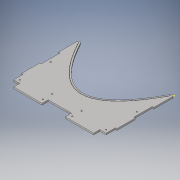
# Autodesk Inventor part: vrRig_v01r1_top
Saved by Autodesk Inventor 2016 (Build 200138000, 138)
## iProperties
Created: 2018-01-13
Part Number: vrRig_v01r1_top
Material: Generic
Document SubType Name: Modeling
Designer: harveylab
Density: 1 g/cm^3
Appearance: Default
Author: harveylab
Autodesk Inventor part; units mm, degrees
ref_plane "YZ Plane" through (0, 0, 0) normal (1, 0, 0) x (0, 1, 0)
ref_plane "XZ Plane" through (0, 0, 0) normal (0, 1, 0) x (-1, 0, 0)
ref_plane "XY Plane" through (0, 0, 0) normal (0, 0, 1) x (1, 0, 0)
sketch "Sketch1" plane through (0, 0, 0) normal (0, 1, 0) x (-1, 0, 0)
  circle A0 centre (374.65, 134.145) radius 3.302 construction
  line L0 (387.3499, 6.3502) -> (384.81, 11.082)
  line L1 (384.81, 11.082) -> (382.27, 15.7505)
  line L2 (382.27, 15.7505) -> (379.73, 20.353)
  line L3 (379.73, 20.353) -> (377.19, 24.8945)
  line L4 (377.19, 24.8945) -> (374.65, 29.37)
  line L5 (374.65, 29.37) -> (372.11, 33.7833)
  line L6 (372.11, 33.7833) -> (369.57, 38.133)
  line L7 (369.57, 38.133) -> (367.03, 42.4193)
  line L8 (367.03, 42.4193) -> (364.49, 46.642)
  line L9 (364.49, 46.642) -> (361.95, 50.8013)
  line L10 (361.95, 50.8013) -> (359.41, 54.897)
  line L11 (359.41, 54.897) -> (356.87, 58.9293)
  line L12 (356.87, 58.9293) -> (354.33, 62.898)
  line L13 (354.33, 62.898) -> (351.79, 66.8033)
  line L14 (351.79, 66.8033) -> (349.25, 70.645)
  line L15 (349.25, 70.645) -> (346.71, 74.4233)
  line L16 (346.71, 74.4233) -> (344.17, 78.138)
  line L17 (344.17, 78.138) -> (341.63, 81.7893)
  line L18 (341.63, 81.7893) -> (339.09, 85.377)
  line L19 (339.09, 85.377) -> (336.55, 88.9025)
  line L20 (336.55, 88.9025) -> (334.01, 92.362)
  line L21 (334.01, 92.362) -> (331.47, 95.7605)
  line L22 (331.47, 95.7605) -> (328.93, 99.093)
  line L23 (328.93, 99.093) -> (326.39, 102.3645)
  line L24 (326.39, 102.3645) -> (323.85, 105.57)
  line L25 (323.85, 105.57) -> (321.31, 108.712)
  line L26 (321.31, 108.712) -> (318.77, 111.793)
  line L27 (318.77, 111.793) -> (316.23, 114.8105)
  line L28 (316.23, 114.8105) -> (313.69, 117.762)
  line L29 (313.69, 117.762) -> (311.15, 120.6525)
  line L30 (311.15, 120.6525) -> (308.61, 123.477)
  line L31 (308.61, 123.477) -> (306.07, 126.2405)
  line L32 (306.07, 126.2405) -> (303.53, 128.938)
  line L33 (303.53, 128.938) -> (300.99, 131.5745)
  line L34 (300.99, 131.5745) -> (298.45, 134.145)
  line L35 (298.45, 134.145) -> (295.91, 136.652)
  line L36 (295.91, 136.652) -> (293.37, 139.098)
  line L37 (293.37, 139.098) -> (290.83, 141.478)
  line L38 (290.83, 141.478) -> (288.29, 143.797)
  line L39 (288.29, 143.797) -> (285.75, 146.0525)
  line L40 (285.75, 146.0525) -> (283.21, 148.242)
  line L41 (283.21, 148.242) -> (280.67, 150.368)
  line L42 (280.67, 150.368) -> (278.13, 152.433)
  line L43 (278.13, 152.433) -> (275.59, 154.4345)
  line L44 (275.59, 154.4345) -> (273.05, 156.37)
  line L45 (273.05, 156.37) -> (270.51, 158.2445)
  line L46 (270.51, 158.2445) -> (267.97, 160.053)
  line L47 (267.97, 160.053) -> (265.43, 161.8005)
  line L48 (265.43, 161.8005) -> (262.89, 163.482)
  line L49 (262.89, 163.482) -> (260.35, 165.1025)
  line L50 (260.35, 165.1025) -> (257.81, 166.657)
  line L51 (257.81, 166.657) -> (255.27, 168.1505)
  line L52 (255.27, 168.1505) -> (252.73, 169.578)
  line L53 (252.73, 169.578) -> (250.19, 170.9445)
  line L54 (250.19, 170.9445) -> (247.65, 172.245)
  line L55 (247.65, 172.245) -> (245.11, 173.4845)
  line L56 (245.11, 173.4845) -> (242.57, 174.658)
  line L57 (242.57, 174.658) -> (240.03, 175.768)
  line L58 (240.03, 175.768) -> (237.49, 176.817)
  line L59 (237.49, 176.817) -> (234.95, 177.8025)
  line L60 (234.95, 177.8025) -> (232.41, 178.722)
  line L61 (232.41, 178.722) -> (229.87, 179.5805)
  line L62 (229.87, 179.5805) -> (227.33, 180.373)
  line L63 (227.33, 180.373) -> (224.79, 181.102)
  line L64 (224.79, 181.102) -> (222.25, 181.77)
  line L65 (222.25, 181.77) -> (219.71, 182.372)
  line L66 (219.71, 182.372) -> (217.17, 182.913)
  line L67 (217.17, 182.913) -> (214.63, 183.388)
  line L68 (214.63, 183.388) -> (212.09, 183.802)
  line L69 (212.09, 183.802) -> (209.55, 184.1525)
  line L70 (209.55, 184.1525) -> (207.01, 184.437)
  line L71 (207.01, 184.437) -> (204.47, 184.658)
  line L72 (204.47, 184.658) -> (201.93, 184.818)
  line L73 (201.93, 184.818) -> (199.39, 184.9145)
  line L74 (199.39, 184.9145) -> (196.85, 184.945)
  line L75 (381.755, 3.3486) -> (379.2235, 8.0648)
  line L76 (379.2235, 8.0648) -> (376.7012, 12.7009)
  line L77 (376.7012, 12.7009) -> (374.1791, 17.2709)
  line L78 (374.1791, 17.2709) -> (371.6575, 21.7794)
  line L79 (371.6575, 21.7794) -> (369.1368, 26.2209)
  line L80 (369.1368, 26.2209) -> (366.6163, 30.6003)
  line L81 (366.6163, 30.6003) -> (364.0967, 34.9152)
  line L82 (364.0967, 34.9152) -> (361.5777, 39.1659)
  line L83 (361.5777, 39.1659) -> (359.0595, 43.3525)
  line L84 (359.0595, 43.3525) -> (356.5419, 47.475)
  line L85 (356.5419, 47.475) -> (354.0252, 51.5332)
  line L86 (354.0252, 51.5332) -> (351.5092, 55.5273)
  line L87 (351.5092, 55.5273) -> (348.9941, 59.4572)
  line L88 (348.9941, 59.4572) -> (346.4798, 63.3229)
  line L89 (346.4798, 63.3229) -> (343.9665, 67.1244)
  line L90 (343.9665, 67.1244) -> (341.454, 70.8616)
  line L91 (341.454, 70.8616) -> (338.9426, 74.5346)
  line L92 (338.9426, 74.5346) -> (336.4321, 78.1433)
  line L93 (336.4321, 78.1433) -> (333.9225, 81.6883)
  line L94 (333.9225, 81.6883) -> (331.4145, 85.1693)
  line L95 (331.4145, 85.1693) -> (328.9074, 88.584)
  line L96 (328.9074, 88.584) -> (326.4015, 91.9369)
  line L97 (326.4015, 91.9369) -> (323.8968, 95.223)
  line L98 (323.8968, 95.223) -> (321.3935, 98.4473)
  line L99 (321.3935, 98.4473) -> (318.8923, 101.6039)
  line L100 (318.8923, 101.6039) -> (316.3909, 104.698)
  line L101 (316.3909, 104.698) -> (313.891, 107.7305)
  line L102 (313.891, 107.7305) -> (311.3942, 110.6966)
  line L103 (311.3942, 110.6966) -> (308.8983, 113.5969)
  line L104 (308.8983, 113.5969) -> (306.404, 116.4354)
  line L105 (306.404, 116.4354) -> (303.9114, 119.2072)
  line L106 (303.9114, 119.2072) -> (301.4206, 121.9171)
  line L107 (301.4206, 121.9171) -> (298.9317, 124.5603)
  line L108 (298.9317, 124.5603) -> (296.4448, 127.1417)
  line L109 (296.4448, 127.1417) -> (293.961, 129.6553)
  line L110 (293.961, 129.6553) -> (291.4771, 132.107)
  line L111 (291.4771, 132.107) -> (288.9965, 134.4958)
  line L112 (288.9965, 134.4958) -> (286.5181, 136.818)
  line L113 (286.5181, 136.818) -> (284.0408, 139.0798)
  line L114 (284.0408, 139.0798) -> (281.5685, 141.2752)
  line L115 (281.5685, 141.2752) -> (279.0989, 143.404)
  line L116 (279.0989, 143.404) -> (276.629, 145.4713)
  line L117 (276.629, 145.4713) -> (274.1617, 147.4772)
  line L118 (274.1617, 147.4772) -> (271.7002, 149.4169)
  line L119 (271.7002, 149.4169) -> (269.2401, 151.2915)
  line L120 (269.2401, 151.2915) -> (266.7828, 153.105)
  line L121 (266.7828, 153.105) -> (264.3286, 154.8524)
  line L122 (264.3286, 154.8524) -> (261.8774, 156.5388)
  line L123 (261.8774, 156.5388) -> (259.4294, 158.1594)
  line L124 (259.4294, 158.1594) -> (256.9846, 159.7192)
  line L125 (256.9846, 159.7192) -> (254.543, 161.2134)
  line L126 (254.543, 161.2134) -> (252.1048, 162.6471)
  line L127 (252.1048, 162.6471) -> (249.6699, 164.0155)
  line L128 (249.6699, 164.0155) -> (247.2384, 165.3236)
  line L129 (247.2384, 165.3236) -> (244.8103, 166.5668)
  line L130 (244.8103, 166.5668) -> (242.3856, 167.7501)
  line L131 (242.3856, 167.7501) -> (239.9667, 168.8676)
  line L132 (239.9667, 168.8676) -> (237.5463, 169.9253)
  line L133 (237.5463, 169.9253) -> (235.1292, 170.9236)
  line L134 (235.1292, 170.9236) -> (232.7205, 171.8582)
  line L135 (232.7205, 171.8582) -> (230.3123, 172.7299)
  line L136 (230.3123, 172.7299) -> (227.9074, 173.5428)
  line L137 (227.9074, 173.5428) -> (225.5082, 174.2913)
  line L138 (225.5082, 174.2913) -> (223.1063, 174.9807)
  line L139 (223.1063, 174.9807) -> (220.71, 175.6109)
  line L140 (220.71, 175.6109) -> (218.3161, 176.1783)
  line L141 (218.3161, 176.1783) -> (215.9247, 176.6876)
  line L142 (215.9247, 176.6876) -> (213.5354, 177.1344)
  line L143 (213.5354, 177.1344) -> (211.145, 177.5241)
  line L144 (211.145, 177.5241) -> (208.7624, 177.8529)
  line L145 (208.7624, 177.8529) -> (206.3813, 178.1196)
  line L146 (206.3813, 178.1196) -> (203.9951, 178.3272)
  line L147 (203.9951, 178.3272) -> (201.6097, 178.4774)
  line L148 (201.6097, 178.4774) -> (199.2313, 178.5678)
  line L149 (199.2313, 178.5678) -> (196.9262, 178.5955)
  line L150 (386.6786, 5.9898) -> (384.1396, 10.72)
  line L151 (384.1396, 10.72) -> (381.6018, 15.3846)
  line L152 (381.6018, 15.3846) -> (379.0639, 19.9832)
  line L153 (379.0639, 19.9832) -> (376.5261, 24.5207)
  line L154 (376.5261, 24.5207) -> (373.9884, 28.9921)
  line L155 (373.9884, 28.9921) -> (371.4508, 33.4013)
  line L156 (371.4508, 33.4013) -> (368.9132, 37.7469)
  line L157 (368.9132, 37.7469) -> (366.3757, 42.0289)
  line L158 (366.3757, 42.0289) -> (363.8384, 46.2473)
  line L159 (363.8384, 46.2473) -> (361.3011, 50.4021)
  line L160 (361.3011, 50.4021) -> (358.7638, 54.4934)
  line L161 (358.7638, 54.4934) -> (356.2267, 58.521)
  line L162 (356.2267, 58.521) -> (353.6897, 62.4851)
  line L163 (353.6897, 62.4851) -> (351.1528, 66.3856)
  line L164 (351.1528, 66.3856) -> (348.616, 70.2225)
  line L165 (348.616, 70.2225) -> (346.0793, 73.9959)
  line L166 (346.0793, 73.9959) -> (343.5427, 77.7056)
  line L167 (343.5427, 77.7056) -> (341.0063, 81.3518)
  line L168 (341.0063, 81.3518) -> (338.4699, 84.9344)
  line L169 (338.4699, 84.9344) -> (335.9338, 88.4545)
  line L170 (335.9338, 88.4545) -> (333.3977, 91.9087)
  line L171 (333.3977, 91.9087) -> (330.8618, 95.3017)
  line L172 (330.8618, 95.3017) -> (328.326, 98.6286)
  line L173 (328.326, 98.6286) -> (325.7904, 101.8945)
  line L174 (325.7904, 101.8945) -> (323.2551, 105.0941)
  line L175 (323.2551, 105.0941) -> (320.7197, 108.2303)
  line L176 (320.7197, 108.2303) -> (318.1845, 111.3055)
  line L177 (318.1845, 111.3055) -> (315.6497, 114.3169)
  line L178 (315.6497, 114.3169) -> (313.115, 117.2622)
  line L179 (313.115, 117.2622) -> (310.5805, 120.1465)
  line L180 (310.5805, 120.1465) -> (308.0462, 122.9646)
  line L181 (308.0462, 122.9646) -> (305.5121, 125.7217)
  line L182 (305.5121, 125.7217) -> (302.9782, 128.4127)
  line L183 (302.9782, 128.4127) -> (300.4446, 131.0426)
  line L184 (300.4446, 131.0426) -> (297.9113, 133.6063)
  line L185 (297.9113, 133.6063) -> (295.3781, 136.1066)
  line L186 (295.3781, 136.1066) -> (292.8452, 138.5457)
  line L187 (292.8452, 138.5457) -> (290.3126, 140.9188)
  line L188 (290.3126, 140.9188) -> (287.7801, 143.2309)
  line L189 (287.7801, 143.2309) -> (285.2482, 145.4793)
  line L190 (285.2482, 145.4793) -> (282.7167, 147.6615)
  line L191 (282.7167, 147.6615) -> (280.1851, 149.7804)
  line L192 (280.1851, 149.7804) -> (277.6538, 151.8383)
  line L193 (277.6538, 151.8383) -> (275.1232, 153.8324)
  line L194 (275.1232, 153.8324) -> (272.5928, 155.7606)
  line L195 (272.5928, 155.7606) -> (270.0628, 157.6278)
  line L196 (270.0628, 157.6278) -> (267.5331, 159.4289)
  line L197 (267.5331, 159.4289) -> (265.0037, 161.1691)
  line L198 (265.0037, 161.1691) -> (262.4747, 162.8433)
  line L199 (262.4747, 162.8433) -> (259.9462, 164.4565)
  line L200 (259.9462, 164.4565) -> (257.418, 166.0038)
  line L201 (257.418, 166.0038) -> (254.8902, 167.4901)
  line L202 (254.8902, 167.4901) -> (252.3628, 168.9105)
  line L203 (252.3628, 168.9105) -> (249.8358, 170.27)
  line L204 (249.8358, 170.27) -> (247.3093, 171.5636)
  line L205 (247.3093, 171.5636) -> (244.7831, 172.7964)
  line L206 (244.7831, 172.7964) -> (242.2576, 173.9632)
  line L207 (242.2576, 173.9632) -> (239.732, 175.0669)
  line L208 (239.732, 175.0669) -> (237.2067, 176.1098)
  line L209 (237.2067, 176.1098) -> (234.6825, 177.0892)
  line L210 (234.6825, 177.0892) -> (232.1583, 178.003)
  line L211 (232.1583, 178.003) -> (229.6345, 178.856)
  line L212 (229.6345, 178.856) -> (227.1114, 179.6432)
  line L213 (227.1114, 179.6432) -> (224.588, 180.3674)
  line L214 (224.588, 180.3674) -> (222.0652, 181.0309)
  line L215 (222.0652, 181.0309) -> (219.5428, 181.6287)
  line L216 (219.5428, 181.6287) -> (217.0206, 182.166)
  line L217 (217.0206, 182.166) -> (214.4987, 182.6376)
  line L218 (214.4987, 182.6376) -> (211.9766, 183.0487)
  line L219 (211.9766, 183.0487) -> (209.4555, 183.3966)
  line L220 (209.4555, 183.3966) -> (206.9346, 183.6789)
  line L221 (206.9346, 183.6789) -> (204.413, 183.8983)
  line L222 (204.413, 183.8983) -> (201.8916, 184.0571)
  line L223 (201.8916, 184.0571) -> (199.371, 184.1529)
  line L224 (199.371, 184.1529) -> (196.8592, 184.1831)
  arc A1 (381.755, 3.3486) -> (393.6991, 6.3502) centre (387.3499, 6.3502) ccw
  line L225 (393.6991, 6.3502) -> (393.6991, 7.1452)
  line L226 (387.3499, 6.3502) -> (386.6786, 5.9898)
  line L227 (393.6991, 7.1452) -> (393.6991, 83.3452)
  line L228 (393.6991, 83.3452) -> (387.3491, 83.3452)
  line L229 (387.3491, 83.3452) -> (387.3491, 159.5452)
  line L230 (387.3491, 159.5452) -> (393.6991, 159.5452)
  line L231 (393.6991, 159.5452) -> (393.6991, 235.745)
  line L232 (393.6991, 235.745) -> (387.35, 235.745)
  line L233 (387.35, 235.745) -> (387.35, 273.845)
  circle A2 centre (19.05, 134.145) radius 3.302 construction
  line L234 (6.35, 6.35) -> (8.89, 11.082)
  line L235 (8.89, 11.082) -> (11.43, 15.7505)
  line L236 (11.43, 15.7505) -> (13.97, 20.353)
  line L237 (13.97, 20.353) -> (16.51, 24.8945)
  line L238 (16.51, 24.8945) -> (19.05, 29.37)
  line L239 (19.05, 29.37) -> (21.59, 33.7833)
  line L240 (21.59, 33.7833) -> (24.13, 38.133)
  line L241 (24.13, 38.133) -> (26.67, 42.4193)
  line L242 (26.67, 42.4193) -> (29.21, 46.642)
  line L243 (29.21, 46.642) -> (31.75, 50.8013)
  line L244 (31.75, 50.8013) -> (34.29, 54.897)
  line L245 (34.29, 54.897) -> (36.83, 58.9293)
  line L246 (36.83, 58.9293) -> (39.37, 62.898)
  line L247 (39.37, 62.898) -> (41.91, 66.8033)
  line L248 (41.91, 66.8033) -> (44.45, 70.645)
  line L249 (44.45, 70.645) -> (46.99, 74.4233)
  line L250 (46.99, 74.4233) -> (49.53, 78.138)
  line L251 (49.53, 78.138) -> (52.07, 81.7893)
  line L252 (52.07, 81.7893) -> (54.61, 85.377)
  line L253 (54.61, 85.377) -> (57.15, 88.9025)
  line L254 (57.15, 88.9025) -> (59.69, 92.362)
  line L255 (59.69, 92.362) -> (62.23, 95.7605)
  line L256 (62.23, 95.7605) -> (64.77, 99.093)
  line L257 (64.77, 99.093) -> (67.31, 102.3645)
  line L258 (67.31, 102.3645) -> (69.85, 105.57)
  line L259 (69.85, 105.57) -> (72.39, 108.712)
  line L260 (72.39, 108.712) -> (74.93, 111.793)
  line L261 (74.93, 111.793) -> (77.47, 114.8105)
  line L262 (77.47, 114.8105) -> (80.01, 117.762)
  line L263 (80.01, 117.762) -> (82.55, 120.6525)
  line L264 (82.55, 120.6525) -> (85.09, 123.477)
  line L265 (85.09, 123.477) -> (87.63, 126.2405)
  line L266 (87.63, 126.2405) -> (90.17, 128.938)
  line L267 (90.17, 128.938) -> (92.71, 131.5745)
  line L268 (92.71, 131.5745) -> (95.25, 134.145)
  line L269 (95.25, 134.145) -> (97.79, 136.652)
  line L270 (97.79, 136.652) -> (100.33, 139.098)
  line L271 (100.33, 139.098) -> (102.87, 141.478)
  line L272 (102.87, 141.478) -> (105.41, 143.797)
  line L273 (105.41, 143.797) -> (107.95, 146.0525)
  line L274 (107.95, 146.0525) -> (110.49, 148.242)
  line L275 (110.49, 148.242) -> (113.03, 150.368)
  line L276 (113.03, 150.368) -> (115.57, 152.433)
  line L277 (115.57, 152.433) -> (118.11, 154.4345)
  line L278 (118.11, 154.4345) -> (120.65, 156.37)
  line L279 (120.65, 156.37) -> (123.19, 158.2445)
  line L280 (123.19, 158.2445) -> (125.73, 160.053)
  line L281 (125.73, 160.053) -> (128.27, 161.8005)
  line L282 (128.27, 161.8005) -> (130.81, 163.482)
  line L283 (130.81, 163.482) -> (133.35, 165.1025)
  line L284 (133.35, 165.1025) -> (135.89, 166.657)
  line L285 (135.89, 166.657) -> (138.43, 168.1505)
  line L286 (138.43, 168.1505) -> (140.97, 169.578)
  line L287 (140.97, 169.578) -> (143.51, 170.9445)
  line L288 (143.51, 170.9445) -> (146.05, 172.245)
  line L289 (146.05, 172.245) -> (148.59, 173.4845)
  line L290 (148.59, 173.4845) -> (151.13, 174.658)
  line L291 (151.13, 174.658) -> (153.67, 175.768)
  line L292 (153.67, 175.768) -> (156.21, 176.817)
  line L293 (156.21, 176.817) -> (158.75, 177.8025)
  line L294 (158.75, 177.8025) -> (161.29, 178.722)
  line L295 (161.29, 178.722) -> (163.83, 179.5805)
  line L296 (163.83, 179.5805) -> (166.37, 180.373)
  line L297 (166.37, 180.373) -> (168.91, 181.102)
  line L298 (168.91, 181.102) -> (171.45, 181.77)
  line L299 (171.45, 181.77) -> (173.99, 182.372)
  line L300 (173.99, 182.372) -> (176.53, 182.913)
  line L301 (176.53, 182.913) -> (179.07, 183.388)
  line L302 (179.07, 183.388) -> (181.61, 183.802)
  line L303 (181.61, 183.802) -> (184.15, 184.1525)
  line L304 (184.15, 184.1525) -> (186.69, 184.437)
  line L305 (186.69, 184.437) -> (189.23, 184.658)
  line L306 (189.23, 184.658) -> (191.77, 184.818)
  line L307 (191.77, 184.818) -> (194.31, 184.9145)
  line L308 (194.31, 184.9145) -> (196.85, 184.945)
  line L309 (11.945, 3.3468) -> (14.4765, 8.063)
  line L310 (14.4765, 8.063) -> (16.9988, 12.699)
  line L311 (16.9988, 12.699) -> (19.5209, 17.2691)
  line L312 (19.5209, 17.2691) -> (22.0424, 21.7776)
  line L313 (22.0424, 21.7776) -> (24.5631, 26.2191)
  line L314 (24.5631, 26.2191) -> (27.0836, 30.5984)
  line L315 (27.0836, 30.5984) -> (29.6033, 34.9133)
  line L316 (29.6033, 34.9133) -> (32.1222, 39.1641)
  line L317 (32.1222, 39.1641) -> (34.6405, 43.3507)
  line L318 (34.6405, 43.3507) -> (37.158, 47.4731)
  line L319 (37.158, 47.4731) -> (39.6748, 51.5314)
  line L320 (39.6748, 51.5314) -> (42.1907, 55.5255)
  line L321 (42.1907, 55.5255) -> (44.7059, 59.4554)
  line L322 (44.7059, 59.4554) -> (47.2201, 63.3211)
  line L323 (47.2201, 63.3211) -> (49.7335, 67.1225)
  line L324 (49.7335, 67.1225) -> (52.2459, 70.8598)
  line L325 (52.2459, 70.8598) -> (54.7574, 74.5328)
  line L326 (54.7574, 74.5328) -> (57.2678, 78.1415)
  line L327 (57.2678, 78.1415) -> (59.7775, 81.6864)
  line L328 (59.7775, 81.6864) -> (62.2854, 85.1675)
  line L329 (62.2854, 85.1675) -> (64.7926, 88.5822)
  line L330 (64.7926, 88.5822) -> (67.2985, 91.9351)
  line L331 (67.2985, 91.9351) -> (69.8031, 95.2212)
  line L332 (69.8031, 95.2212) -> (72.3065, 98.4455)
  line L333 (72.3065, 98.4455) -> (74.8077, 101.602)
  line L334 (74.8077, 101.602) -> (77.3091, 104.6962)
  line L335 (77.3091, 104.6962) -> (79.809, 107.7286)
  line L336 (79.809, 107.7286) -> (82.3057, 110.6947)
  line L337 (82.3057, 110.6947) -> (84.8017, 113.5951)
  line L338 (84.8017, 113.5951) -> (87.296, 116.4336)
  line L339 (87.296, 116.4336) -> (89.7886, 119.2053)
  line L340 (89.7886, 119.2053) -> (92.2793, 121.9153)
  line L341 (92.2793, 121.9153) -> (94.7682, 124.5585)
  line L342 (94.7682, 124.5585) -> (97.2551, 127.1399)
  line L343 (97.2551, 127.1399) -> (99.7389, 129.6535)
  line L344 (99.7389, 129.6535) -> (102.2229, 132.1051)
  line L345 (102.2229, 132.1051) -> (104.7035, 134.494)
  line L346 (104.7035, 134.494) -> (107.1818, 136.8162)
  line L347 (107.1818, 136.8162) -> (109.6591, 139.078)
  line L348 (109.6591, 139.078) -> (112.1314, 141.2733)
  line L349 (112.1314, 141.2733) -> (114.6011, 143.4022)
  line L350 (114.6011, 143.4022) -> (117.0709, 145.4695)
  line L351 (117.0709, 145.4695) -> (119.5382, 147.4754)
  line L352 (119.5382, 147.4754) -> (121.9997, 149.415)
  line L353 (121.9997, 149.415) -> (124.4599, 151.2897)
  line L354 (124.4599, 151.2897) -> (126.9171, 153.1031)
  line L355 (126.9171, 153.1031) -> (129.3714, 154.8506)
  line L356 (129.3714, 154.8506) -> (131.8225, 156.5369)
  line L357 (131.8225, 156.5369) -> (134.2706, 158.1575)
  line L358 (134.2706, 158.1575) -> (136.7154, 159.7173)
  line L359 (136.7154, 159.7173) -> (139.1569, 161.2116)
  line L360 (139.1569, 161.2116) -> (141.5952, 162.6452)
  line L361 (141.5952, 162.6452) -> (144.0301, 164.0137)
  line L362 (144.0301, 164.0137) -> (146.4616, 165.3218)
  line L363 (146.4616, 165.3218) -> (148.8897, 166.565)
  line L364 (148.8897, 166.565) -> (151.3144, 167.7483)
  line L365 (151.3144, 167.7483) -> (153.7333, 168.8658)
  line L366 (153.7333, 168.8658) -> (156.1536, 169.9235)
  line L367 (156.1536, 169.9235) -> (158.5707, 170.9218)
  line L368 (158.5707, 170.9218) -> (160.9795, 171.8563)
  line L369 (160.9795, 171.8563) -> (163.3876, 172.7281)
  line L370 (163.3876, 172.7281) -> (165.7926, 173.541)
  line L371 (165.7926, 173.541) -> (168.1918, 174.2895)
  line L372 (168.1918, 174.2895) -> (170.5937, 174.9789)
  line L373 (170.5937, 174.9789) -> (172.99, 175.6091)
  line L374 (172.99, 175.6091) -> (175.3838, 176.1764)
  line L375 (175.3838, 176.1764) -> (177.7753, 176.6858)
  line L376 (177.7753, 176.6858) -> (180.1646, 177.1326)
  line L377 (180.1646, 177.1326) -> (182.555, 177.5222)
  line L378 (182.555, 177.5222) -> (184.9376, 177.851)
  line L379 (184.9376, 177.851) -> (187.3187, 178.1177)
  line L380 (187.3187, 178.1177) -> (189.7049, 178.3253)
  line L381 (189.7049, 178.3253) -> (192.0903, 178.4756)
  line L382 (192.0903, 178.4756) -> (194.4687, 178.566)
  line L383 (194.4687, 178.566) -> (196.9262, 178.5955)
  line L384 (7.0214, 5.9896) -> (9.5604, 10.7197)
  line L385 (9.5604, 10.7197) -> (12.0983, 15.3844)
  line L386 (12.0983, 15.3844) -> (14.6361, 19.9829)
  line L387 (14.6361, 19.9829) -> (17.1739, 24.5205)
  line L388 (17.1739, 24.5205) -> (19.7116, 28.9919)
  line L389 (19.7116, 28.9919) -> (22.2492, 33.4011)
  line L390 (22.2492, 33.4011) -> (24.7868, 37.7467)
  line L391 (24.7868, 37.7467) -> (27.3243, 42.0286)
  line L392 (27.3243, 42.0286) -> (29.8617, 46.2471)
  line L393 (29.8617, 46.2471) -> (32.399, 50.4019)
  line L394 (32.399, 50.4019) -> (34.9362, 54.4931)
  line L395 (34.9362, 54.4931) -> (37.4733, 58.5208)
  line L396 (37.4733, 58.5208) -> (40.0103, 62.4849)
  line L397 (40.0103, 62.4849) -> (42.5472, 66.3854)
  line L398 (42.5472, 66.3854) -> (45.084, 70.2223)
  line L399 (45.084, 70.2223) -> (47.6207, 73.9956)
  line L400 (47.6207, 73.9956) -> (50.1573, 77.7054)
  line L401 (50.1573, 77.7054) -> (52.6937, 81.3515)
  line L402 (52.6937, 81.3515) -> (55.2301, 84.9341)
  line L403 (55.2301, 84.9341) -> (57.7663, 88.4543)
  line L404 (57.7663, 88.4543) -> (60.3023, 91.9084)
  line L405 (60.3023, 91.9084) -> (62.8382, 95.3015)
  line L406 (62.8382, 95.3015) -> (65.374, 98.6284)
  line L407 (65.374, 98.6284) -> (67.9096, 101.8942)
  line L408 (67.9096, 101.8942) -> (70.4449, 105.0939)
  line L409 (70.4449, 105.0939) -> (72.9803, 108.2301)
  line L410 (72.9803, 108.2301) -> (75.5155, 111.3053)
  line L411 (75.5155, 111.3053) -> (78.0503, 114.3166)
  line L412 (78.0503, 114.3166) -> (80.585, 117.262)
  line L413 (80.585, 117.262) -> (83.1195, 120.1463)
  line L414 (83.1195, 120.1463) -> (85.6538, 122.9644)
  line L415 (85.6538, 122.9644) -> (88.1879, 125.7215)
  line L416 (88.1879, 125.7215) -> (90.7218, 128.4125)
  line L417 (90.7218, 128.4125) -> (93.2554, 131.0424)
  line L418 (93.2554, 131.0424) -> (95.7887, 133.606)
  line L419 (95.7887, 133.606) -> (98.322, 136.1064)
  line L420 (98.322, 136.1064) -> (100.8548, 138.5455)
  line L421 (100.8548, 138.5455) -> (103.3874, 140.9186)
  line L422 (103.3874, 140.9186) -> (105.9199, 143.2307)
  line L423 (105.9199, 143.2307) -> (108.4518, 145.479)
  line L424 (108.4518, 145.479) -> (110.9833, 147.6612)
  line L425 (110.9833, 147.6612) -> (113.5149, 149.7802)
  line L426 (113.5149, 149.7802) -> (116.0462, 151.8381)
  line L427 (116.0462, 151.8381) -> (118.5768, 153.8322)
  line L428 (118.5768, 153.8322) -> (121.1072, 155.7604)
  line L429 (121.1072, 155.7604) -> (123.6373, 157.6276)
  line L430 (123.6373, 157.6276) -> (126.167, 159.4287)
  line L431 (126.167, 159.4287) -> (128.6963, 161.1689)
  line L432 (128.6963, 161.1689) -> (131.2253, 162.8431)
  line L433 (131.2253, 162.8431) -> (133.7539, 164.4563)
  line L434 (133.7539, 164.4563) -> (136.282, 166.0036)
  line L435 (136.282, 166.0036) -> (138.8098, 167.4899)
  line L436 (138.8098, 167.4899) -> (141.3372, 168.9103)
  line L437 (141.3372, 168.9103) -> (143.8642, 170.2698)
  line L438 (143.8642, 170.2698) -> (146.3908, 171.5634)
  line L439 (146.3908, 171.5634) -> (148.9169, 172.7962)
  line L440 (148.9169, 172.7962) -> (151.4424, 173.9629)
  line L441 (151.4424, 173.9629) -> (153.968, 175.0667)
  line L442 (153.968, 175.0667) -> (156.4933, 176.1096)
  line L443 (156.4933, 176.1096) -> (159.0176, 177.089)
  line L444 (159.0176, 177.089) -> (161.5417, 178.0027)
  line L445 (161.5417, 178.0027) -> (164.0655, 178.8558)
  line L446 (164.0655, 178.8558) -> (166.5886, 179.643)
  line L447 (166.5886, 179.643) -> (169.112, 180.3672)
  line L448 (169.112, 180.3672) -> (171.6348, 181.0307)
  line L449 (171.6348, 181.0307) -> (174.1573, 181.6285)
  line L450 (174.1573, 181.6285) -> (176.6794, 182.1657)
  line L451 (176.6794, 182.1657) -> (179.2014, 182.6373)
  line L452 (179.2014, 182.6373) -> (181.7234, 183.0484)
  line L453 (181.7234, 183.0484) -> (184.2445, 183.3964)
  line L454 (184.2445, 183.3964) -> (186.7655, 183.6787)
  line L455 (186.7655, 183.6787) -> (189.287, 183.8981)
  line L456 (189.287, 183.8981) -> (191.8084, 184.0569)
  line L457 (191.8084, 184.0569) -> (194.3291, 184.1527)
  line L458 (194.3291, 184.1527) -> (196.8592, 184.1831)
  arc A3 (0, 6.35) -> (11.945, 3.3468) centre (6.35, 6.35) ccw
  line L459 (0, 6.35) -> (0, 7.145)
  line L460 (6.35, 6.35) -> (7.0214, 5.9896)
  line L461 (0, 7.145) -> (0, 83.345)
  line L462 (0, 83.345) -> (6.35, 83.345)
  line L463 (6.35, 83.345) -> (6.35, 159.545)
  line L464 (6.35, 159.545) -> (0, 159.545)
  line L465 (0, 159.545) -> (0, 235.745)
  line L466 (0, 235.745) -> (6.35, 235.745)
  line L467 (6.35, 235.745) -> (6.35, 273.845)
  circle A4 centre (257.3579, 283.2837) radius 2.54 construction
  circle A5 centre (257.3579, 245.1837) radius 2.54 construction
  circle A6 centre (136.3421, 283.2837) radius 2.54 construction
  circle A7 centre (136.3421, 245.1837) radius 2.54 construction
  line L468 (244.6579, 299.245) -> (244.6579, 273.845)
  line L469 (244.6579, 273.845) -> (196.85, 273.845)
  line L470 (149.0421, 299.245) -> (149.0421, 273.845)
  line L471 (149.0421, 273.845) -> (196.85, 273.845)
  line L472 (149.0421, 299.245) -> (31.75, 299.245)
  line L473 (244.6579, 299.245) -> (361.95, 299.245)
  circle A8 centre (19.05, 261.145) radius 3.302 construction
  line L474 (6.35, 273.845) -> (31.75, 273.845)
  line L475 (31.75, 273.845) -> (31.75, 299.245)
  line L476 (361.95, 299.245) -> (361.95, 273.845)
  line L477 (361.95, 273.845) -> (387.35, 273.845)
  circle A9 centre (374.65, 261.145) radius 3.302 construction
  point P0 (0, 0)
  constraints: 956 end point, 10 centre point, 8 coincident, 4 point on circle, 4 point on line
sketch "Sketch4" plane through (0, 0, 0) normal (0, 1, 0) x (-1, 0, 0)
  point P0 (0, 0)
  point P1 (19.05, 261.145)
  point P2 (19.05, 134.145)
  point P3 (136.3421, 283.2837)
  point P4 (136.3421, 245.1837)
  point P5 (257.3579, 283.2837)
  point P6 (257.3579, 245.1837)
  point P7 (374.65, 261.145)
  point P8 (374.65, 134.145)
extrude "Extrusion3" add sketch "Sketch1" along normal blind 6.35
hole "Hole1" at (-19.05, 0, 261.145) at (-19.05, 0, 134.145) at (-136.3421, 0, 283.2837) at (-136.3421, 0, 245.1837) at (-257.3579, 0, 283.2837) at (-257.3579, 0, 245.1837) at (-374.65, 0, 261.145) at (-374.65, 0, 134.145) direction (0, 1, 0) diameter 4.9784 depth 19.05 tip angle 118 thread size "1/4-20 UNC" class "2B" standard "ANSI Unified Screw Threads"
sketch "Sketch5" plane through (0, 6.35, 0) normal (0, 1, 0) x (1, 0, 0)
  point P0 (0, 0)
body "Solid3"
